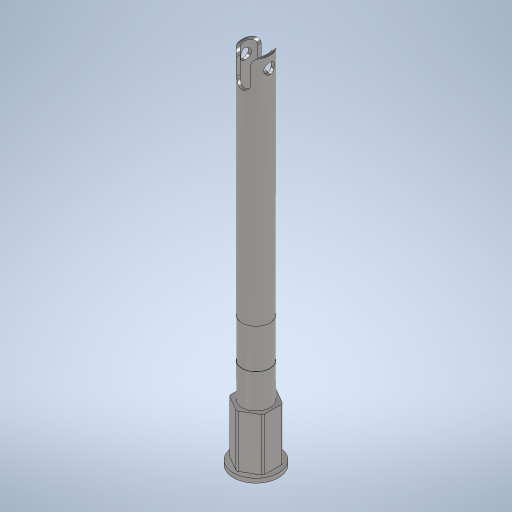
# Autodesk Inventor part: Slider
Saved by Autodesk Inventor 2023.2 (Build 272271000, 271)
## iProperties
Created: 2024-02-03
Part Number: Slider
Material: Stainless Steel
Document SubType Name: Modeling
Designer: Nathan Cai
Mass: 15.7694 g
Surface Area: 47.0442 cm^2
Volume: 1.97118 cm^3
Density: 8 g/cm^3
Appearance: Semi-Polished
Author: Nathan Cai
Autodesk Inventor part; units mm, degrees
ref_plane "YZ Plane" through (0, 0, 0) normal (1, 0, 0) x (0, 1, 0)
ref_plane "XZ Plane" through (0, 0, 0) normal (0, 1, 0) x (-1, 0, 0)
sketch "Sketch1" plane through (0, 0, 0) normal (0, 1, 0) x (-1, 0, 0)
  circle A0 centre (0, 0) radius 3.175
  circle A1 centre (0, 0) radius 4.7625 construction
  circle A2 centre (0, 0) radius 7.9375 construction
  line L0 (0, 0) -> (4.7625, 0) construction
  line L1 (4.7625, -2.7496) -> (0, -5.4993)
  line L2 (0, -5.4993) -> (-4.7625, -2.7496)
  line L3 (-4.7625, -2.7496) -> (-4.7625, 2.7496)
  line L4 (-4.7625, 2.7496) -> (0, 5.4993)
  line L5 (0, 5.4993) -> (4.7625, 2.7496)
  line L6 (4.7625, 2.7496) -> (4.7625, -2.7496)
  arc A3 (4.4712, 0.9165) -> (4.1799, 0) centre (5.7674, 0) ccw
  line L7 (4.7625, 2.7496) -> (0, 0) construction
  arc A4 (4.4712, 0.9165) -> (4.5498, 2.6268) centre (3.175, 1.8331) ccw
  arc A5 (4.1799, 0) -> (4.4712, -0.9165) centre (5.7674, 0) ccw
  arc A6 (4.5498, -2.6268) -> (4.4712, -0.9165) centre (3.175, -1.8331) ccw
  arc A7 (4.5498, 2.6268) -> (3.0293, 3.4139) centre (3.175, 1.8331) ccw
  arc A8 (2.0899, 3.6199) -> (3.0293, 3.4139) centre (2.8837, 4.9947) ccw
  arc A9 (1.4418, 4.3304) -> (2.0899, 3.6199) centre (2.8837, 4.9947) ccw
  arc A10 (1.4418, 4.3304) -> (0, 5.2537) centre (0, 3.6662) ccw
  arc A11 (0, 5.2537) -> (-1.4418, 4.3304) centre (0, 3.6662) ccw
  arc A12 (-2.0899, 3.6199) -> (-1.4418, 4.3304) centre (-2.8837, 4.9947) ccw
  arc A13 (-3.0293, 3.4139) -> (-2.0899, 3.6199) centre (-2.8837, 4.9947) ccw
  arc A14 (-3.0293, 3.4139) -> (-4.5498, 2.6268) centre (-3.175, 1.8331) ccw
  arc A15 (-4.5498, 2.6268) -> (-4.4712, 0.9165) centre (-3.175, 1.8331) ccw
  arc A16 (-4.1799, 0) -> (-4.4712, 0.9165) centre (-5.7674, 0) ccw
  arc A17 (-4.4712, -0.9165) -> (-4.1799, 0) centre (-5.7674, 0) ccw
  arc A18 (-4.4712, -0.9165) -> (-4.5498, -2.6268) centre (-3.175, -1.8331) ccw
  arc A19 (-4.5498, -2.6268) -> (-3.0293, -3.4139) centre (-3.175, -1.8331) ccw
  arc A20 (-2.0899, -3.6199) -> (-3.0293, -3.4139) centre (-2.8837, -4.9947) ccw
  arc A21 (-1.4418, -4.3304) -> (-2.0899, -3.6199) centre (-2.8837, -4.9947) ccw
  arc A22 (-1.4418, -4.3304) -> (0, -5.2537) centre (0, -3.6662) ccw
  arc A23 (0, -5.2537) -> (1.4418, -4.3304) centre (0, -3.6662) ccw
  arc A24 (2.0899, -3.6199) -> (1.4418, -4.3304) centre (2.8837, -4.9947) ccw
  arc A25 (3.0293, -3.4139) -> (2.0899, -3.6199) centre (2.8837, -4.9947) ccw
  arc A26 (3.0293, -3.4139) -> (4.5498, -2.6268) centre (3.175, -1.8331) ccw
  point P0 (2.3813, -4.1244)
  point P1 (4.7625, 1.8331)
  point P2 (3.9688, 3.2079)
  point P3 (0.7938, 5.041)
  point P4 (-0.7937, 5.041)
  point P5 (-3.9687, 3.2079)
  point P6 (-4.7625, 1.8331)
  point P7 (-4.7625, -1.8331)
  point P8 (-3.9688, -3.2079)
  point P9 (-0.7938, -5.041)
  point P10 (0.7937, -5.041)
  point P11 (3.9688, -3.2079)
  point P12 (4.7625, -1.8331)
  dimension "d0" = 6.35
  dimension "d1" = 9.525
  dimension "d2" = 15.875
  dimension "d30" = 1.5875
  dimension "d31" = 1.5875
  dimension "d34" = 360
  constraints: 48 point on circle, 27 centre point, 16 end point, 4 coincident, 4 tangent, 3 point on line, 3 symmetric about line, 1 horizontal, 1 midpoint, 88 other
  measures "d0" diameter of A0
  measures "d1" diameter of A1
  measures "d2" diameter of A2
  measures "d30" radius of A3
  measures "d31" radius of A4
extrude "Extrusion1" add sketch "Sketch1" along normal blind 15.875
sketch "Sketch2" plane through (0, 0, 0) normal (0, -1, 0) x (1, 0, 0)
  circle A0 centre (0, 0) radius 3.175 projected
  circle A1 centre (0, 0) radius 6.35
  dimension "d26" = 12.7
  constraints: 1 centre point, 1 coincident
  measures "d26" diameter of A1
extrude "Extrusion2" add sketch "Sketch2" against normal blind 1.1906
sketch "Sketch3" plane through (0, 0, 0) normal (0, -1, 0) x (1, 0, 0)
  circle A0 centre (0, 0) radius 3.175 projected
  circle A1 centre (0, 0) radius 3.9688
  dimension "d40" = 7.9375
  constraints: 1 centre point, 1 coincident
  measures "d40" diameter of A1
extrude "Extrusion3" add sketch "Sketch3" against normal blind 101.6
thicken "Thicken3" operation cut thickness 0.0254 both sides no extend neighbours yes toward (-0.9967573, 0, 0.0804666) faces at (3.9559, 73.025, -0.3194)
sketch "Sketch5" plane through (0, 0, 0) normal (1, 0, 0) x (0, 1, 0)
  line L0 (0, 0) -> (101.6, 0) construction
  line L1 (101.6, -3.9434) -> (101.6, 3.9434) projected
  circle A0 centre (98.425, 0) radius 1.5
  line L2 (0, 6.35) -> (0, -6.35) projected
  dimension "d47" = 3
  dimension "d56" = 3.175
  constraints: 2 end point, 1 centre point, 1 midpoint, 1 point on line
  measures "d47" diameter of A0
  measures "d56" distance from line of L1 A0.centre
extrude "Extrusion5" cut sketch "Sketch5" along normal through all both and the other way through all
sketch "Sketch6" plane through (0, 0, 0) normal (0, 0, 1) x (1, 0, 0)
  line L0 (0, 107.95) -> (0, 95.25) construction
  line L1 (3.9434, 101.6) -> (-3.9434, 101.6) projected
  line L2 (-1.9844, 107.95) -> (-1.9844, 95.25)
  line L3 (1.9844, 95.25) -> (1.9844, 107.95)
  arc A0 (1.9844, 107.95) -> (-1.9844, 107.95) centre (0, 107.95) ccw
  arc A1 (-1.9844, 95.25) -> (1.9844, 95.25) centre (0, 95.25) ccw
  point P0 (0, 0)
  point P1 (0, 101.6)
  dimension "d51" = 6.35
  dimension "d52" = 3.9688
  constraints: 8 end point, 4 point on circle, 4 tangent, 2 centre point, 2 midpoint, 1 parallel, 1 vertical
  measures "d51" distance of point (0, 101.6) L0.end
  measures "d52" diameter of A1
extrude "Extrusion6" cut sketch "Sketch6" along normal through all both and the other way through all
fillet "Fillet2" radius 1.5875 4 edges at (1.9844, 101.6, -2.9431) (1.9844, 101.6, 2.9431) (-1.9844, 101.6, 2.9431) (-1.9844, 101.6, -2.9431)
chamfer "Chamfer1" distance 0.5 angle 45 1 edges at (3.175, 0, 0)
ref_plane "Work Plane1" through (0, 25.4, 0) normal (0, -1, 0) x (1, 0, 0)
sketch "Sketch7" plane through (0, 25.4, 0) normal (0, -1, 0) x (1, 0, 0)
  circle A0 centre (0, 0) radius 3.9434 projected
  arc A1 (-3.5719, 1.6708) -> (-3.5719, -1.6708) centre (0, 0) ccw projected
  arc A2 (3.5719, -1.6708) -> (3.5719, 1.6708) centre (0, 0) ccw projected
  circle A3 centre (0, 0) radius 3.8925
  point P0 (3.6469, -1.5)
  point P1 (-3.6469, -1.5)
  dimension "d61" = 0.0508
  constraints: 2 horizontal alignment, 1 centre point, 4 other
  measures "d61" radial gap between concentric circles of A0 A3
extrude "Extrusion7" cut sketch "Sketch7" against normal blind 11.1125
fillet "Fillet3" radius 0.75 6 edges at (0, 8.5328, -5.4993) (4.7625, 8.5328, -2.7496) (4.7625, 8.5328, 2.7496) (0, 8.5328, 5.4993) (-4.7625, 8.5328, -2.7496) (-4.7625, 8.5328, 2.7496)
body "Solid1"
